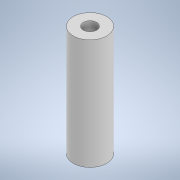
# Autodesk Inventor part: PiMount_spaced_fr
Saved by Autodesk Inventor 2022 (Build 260153000, 153)
## iProperties
Created: 2023-01-04
Part Number: PiMount_spaced_fr
Material: Generic
Document SubType Name: Modeling
Designer: Harmonic Ash
Density: 1 g/cm^3
Appearance: Default
Author: Harmonic Ash
Autodesk Inventor part; units mm, degrees
ref_plane "YZ Plane" through (0, 0, 0) normal (1, 0, 0) x (0, 1, 0)
ref_plane "XZ Plane" through (0, 0, 0) normal (0, 1, 0) x (-1, 0, 0)
ref_plane "XY Plane" through (0, 0, 0) normal (0, 0, 1) x (1, 0, 0)
sketch "Sketch1" plane through (0, 0, 0) normal (0, 0, 1) x (1, 0, 0)
  line L0 (0, 0) -> (0, 16.5)
  line L1 (0, 16.5) -> (-1, 16.5)
  line L2 (-1, 16.5) -> (-1, 0)
  line L3 (-1, 0) -> (0, 0)
  line L4 (-1, 0) -> (-2.5, 0)
  line L5 (-2.5, 0) -> (-2.5, 16.5)
  line L6 (-2.5, 16.5) -> (-1, 16.5)
  dimension "d0" = 16.5
  dimension "d1" = 1
  dimension "d2" = 1.5
  constraints: 14 end point, 4 perpendicular, 2 point on line, 1 parallel, 1 vertical
  measures "d0" distance of L0.start L0.end
  measures "d1" distance of L0.end L1.end
  measures "d2" distance of L2.end L4.end
revolve "Revolution1" add sketch "Sketch1" angle 360 about axis through (0, 0, 0) along (0, 1, 0) contours L4 L5 L6 L2
body "Solid1"
